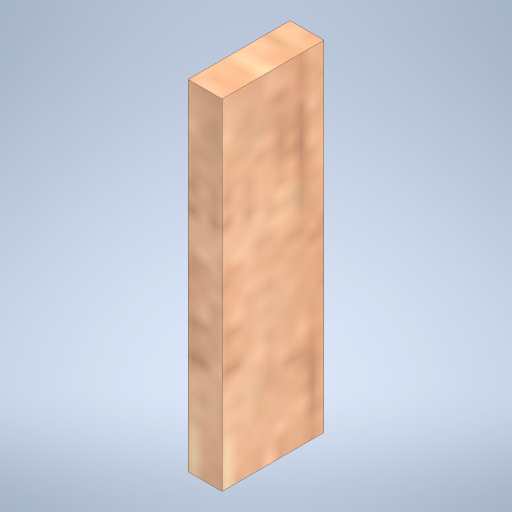
# Autodesk Inventor part: Projectile Launcher Partial Popsicle Stick
Saved by Autodesk Inventor 2024 (Build 280153000, 153)
## iProperties
Created: 2023-09-26
Part Number: Projectile Launcher Partial Popsicle Stick
Material: Wood (Birch)
Document SubType Name: Modeling
Designer: Nick
Density: 0.55 g/cm^3
Appearance: Birch - Natural Polished
Author: Nick
Autodesk Inventor part; units mm, degrees
ref_plane "YZ Plane" through (0, 0, 0) normal (1, 0, 0) x (0, 1, 0)
ref_plane "XZ Plane" through (0, 0, 0) normal (0, 1, 0) x (-1, 0, 0)
ref_plane "XY Plane" through (0, 0, 0) normal (0, 0, 1) x (1, 0, 0)
sketch "Sketch1" plane through (0, 0, 0) normal (0, 1, 0) x (-1, 0, 0)
  line L0 (0, 0) -> (3.175, 0)
  line L1 (3.175, 0) -> (3.175, -9.525)
  line L2 (3.175, -9.525) -> (0, -9.525)
  line L3 (0, -9.525) -> (0, 0)
  dimension "d0" = 3.175
  dimension "d1" = 9.525
  constraints: 8 end point, 2 parallel, 1 horizontal, 1 perpendicular
  measures "d0" distance of L1.end L2.end
  measures "d1" distance of L0.end L1.end
extrude "Extrusion1" add sketch "Sketch1" along normal blind 31.75
body "Solid1"
